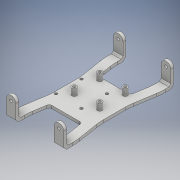
# Autodesk Inventor part: IMU_holder
Saved by Autodesk Inventor 2018 (Build 220112000, 112)
## iProperties
Created: 2018-07-18
Part Number: IMU_holder
Material: Generic
Document SubType Name: Modeling
Designer: Tsche
Density: 1 g/cm^3
Appearance: Default
Author: Tsche
Autodesk Inventor part; units mm, degrees
note: some values were not read from the file. Chosen so that the rebuilt part matches the saved one: direction of "Hole1".
ref_plane "YZ Plane" through (0, 0, 0) normal (1, 0, 0) x (0, 1, 0)
ref_plane "XZ Plane" through (0, 0, 0) normal (0, 1, 0) x (-1, 0, 0)
ref_plane "XY Plane" through (0, 0, 0) normal (0, 0, 1) x (1, 0, 0)
sketch "Sketch1" plane through (0, 0, 0) normal (0, 0, 1) x (1, 0, 0)
  line L0 (-22.86, 13.96) -> (3.81, 13.96) construction
  line L1 (3.81, 13.96) -> (3.81, -12.71) construction
  line L2 (3.81, -12.71) -> (-22.86, -12.71) construction
  line L3 (-22.86, -12.71) -> (-22.86, 13.96) construction
  line L4 (3.81, 0) -> (0, 0) construction
  line L5 (0, 0) -> (0, 13.96) construction
  circle A0 centre (-22.86, 13.96) radius 1.4
  circle A1 centre (3.81, 13.96) radius 1.4
  circle A2 centre (-22.86, -12.71) radius 1.4
  circle A3 centre (3.81, -12.71) radius 1.4
  line L6 (13.96, 22.86) -> (13.96, -3.81) construction
  line L7 (13.96, -3.81) -> (-12.71, -3.81) construction
  line L8 (-12.71, -3.81) -> (-12.71, 22.86) construction
  line L9 (-12.71, 22.86) -> (13.96, 22.86) construction
  line L10 (0, -3.81) -> (0, 0) construction
  line L11 (0, 0) -> (13.96, 0) construction
  circle A4 centre (13.96, 22.86) radius 1.4
  circle A5 centre (13.96, -3.81) radius 1.4
  circle A6 centre (-12.71, 22.86) radius 1.4
  circle A7 centre (-12.71, -3.81) radius 1.4
  line L12 (-30, -57.5) -> (-20, -57.5)
  line L13 (-25, -57.5) -> (-25, -66.2075) construction
  line L14 (25, -57.5) -> (25, -66.2075) construction
  line L15 (0, 215.5444) -> (0, -197.4509) construction
  line L16 (-25.36, 15.21) -> (-25.36, -15.21)
  line L17 (-16.9679, 25.36) -> (16.9679, 25.36)
  line L18 (-30, -57.5) -> (-30, -54.5)
  line L19 (-30, -54.5) -> (30, -54.5) construction
  line L20 (30, -54.5) -> (30, -57.5)
  line L21 (-30, -54.5) -> (-30, -44.5)
  line L22 (-30, -44.5) -> (-25.36, -15.21)
  line L23 (30, -54.5) -> (30, -44.5)
  line L24 (30, -44.5) -> (25.36, -15.21)
  line L25 (25.36, 15.21) -> (25.36, -15.21)
  line L26 (-42, 0) -> (42, 0) construction
  line L27 (-30, 57.5) -> (-20, 57.5)
  line L28 (-25, 57.5) -> (-25, 66.2075) construction
  line L29 (25, 57.5) -> (25, 66.2075) construction
  line L30 (-30, 57.5) -> (-30, 54.5)
  line L31 (-30, 54.5) -> (30, 54.5) construction
  line L32 (30, 54.5) -> (30, 57.5)
  line L33 (-30, 54.5) -> (-30, 44.5)
  line L34 (-30, 44.5) -> (-25.36, 15.21)
  line L35 (30, 44.5) -> (25.36, 15.21)
  line L36 (30, 54.5) -> (30, 44.5)
  line L37 (-16.9679, 25.36) -> (-20, 44.5)
  line L38 (-20, 44.5) -> (-20, 54.5)
  line L39 (16.9679, 25.36) -> (20, 44.5)
  line L40 (20, 44.5) -> (20, 54.5)
  line L41 (0, -215.5444) -> (0, 197.4509) construction
  line L42 (-16.9679, -25.36) -> (16.9679, -25.36)
  line L43 (-16.9679, -25.36) -> (-20, -44.5)
  line L44 (-20, -44.5) -> (-20, -54.5)
  line L45 (16.9679, -25.36) -> (20, -44.5)
  line L46 (20, -44.5) -> (20, -54.5)
  line L47 (-20, -54.5) -> (-20, -57.5)
  line L48 (20, -54.5) -> (20, -57.5)
  line L49 (-20, 54.5) -> (-20, 57.5)
  line L50 (20, 54.5) -> (20, 57.5)
  line L51 (-20, -57.5) -> (20, -57.5) construction
  line L52 (20, -57.5) -> (30, -57.5)
  line L53 (-20, 57.5) -> (20, 57.5) construction
  line L54 (20, 57.5) -> (30, 57.5)
  dimension "d0" = 26.67
  dimension "d1" = 13.96
  dimension "d2" = 3.81
  dimension "d3" = 2.8
  dimension "d6" = 90
  dimension "d8" = 57.5
  dimension "d10" = 50
  dimension "d11" = 5
  dimension "d12" = 2.5
  dimension "d13" = 2.5
  dimension "d16" = 3
  dimension "d17" = 2.5
  dimension "d18" = 10
  dimension "d19" = 10
  dimension "d35" = 5
  constraints: 106 end point, 28 symmetric about line, 13 point on line, 11 coincident, 11 perpendicular, 8 centre point, 7 horizontal, 5 vertical, 4 midpoint, 3 equal radius, 3 parallel, 23 other
  measures "d0" distance of L2.end L0.start
  measures "d1" distance of L4.end L5.end
  measures "d2" distance of L4.start L4.end
  measures "d3" diameter of A0
  measures "d8" distance from line of point (0, 0) L12
  measures "d10" distance between parallel lines of L13 L14
  measures "d11" distance from line of L20.end L14
  measures "d12" distance between parallel lines of L16 L3
  measures "d13" distance from line of L6.start L17
  measures "d16" distance of L12.start L18.end
  measures "d17" horizontal distance of L2.end L16.end
  measures "d18" distance of L18.end L21.end
  measures "d19" distance of L37.end L38.end
  measures "d35" distance between parallel lines of L13 L44
extrude "Extrusion1" add sketch "Sketch1" along normal blind 3
sketch "Sketch2" plane through (0, 0, 3) normal (0, 0, 1) x (1, 0, 0)
  circle A0 centre (-22.86, 13.96) radius 1.4 projected
  circle A1 centre (-12.71, 22.86) radius 1.4 projected
  circle A2 centre (3.81, 13.96) radius 1.4 projected
  circle A3 centre (13.96, 22.86) radius 1.4 projected
  circle A4 centre (13.96, -3.81) radius 1.4 projected
  circle A5 centre (3.81, -12.71) radius 1.4 projected
  circle A6 centre (-12.71, -3.81) radius 1.4 projected
  circle A7 centre (-22.86, -12.71) radius 1.4 projected
  circle A8 centre (-22.86, 13.96) radius 2.5
  line L0 (-25.36, 15.21) -> (-25.36, -15.21) construction
  circle A9 centre (-22.86, -12.71) radius 2.5
  circle A10 centre (-12.71, -3.81) radius 2.5
  circle A11 centre (-12.71, 22.86) radius 2.5
  circle A12 centre (3.81, 13.96) radius 2.5
  circle A13 centre (13.96, 22.86) radius 1.4 projected
  circle A14 centre (13.96, 22.86) radius 2.5
  circle A15 centre (13.96, -3.81) radius 2.5
  circle A16 centre (3.81, -12.71) radius 2.5
  point P0 (0, 0)
  constraints: 8 centre point, 8 coincident, 6 equal radius, 2 tangent
extrude "Extrusion2" add sketch "Sketch2" along normal blind 7 contours A10 | A11 | A14 | A15
sketch "Sketch3" plane through (0, 0, 3) normal (0, 0, 1) x (1, 0, 0)
  line L0 (-30, -54.5) -> (30, -54.5) construction
  line L1 (-30, -57.5) -> (-20, -57.5) construction
  line L2 (-20, -54.5) -> (-20, -57.5) construction
  line L3 (-30, -44.5) -> (-30, -57.5) construction
  line L4 (30, -57.5) -> (30, -44.5) construction
  line L5 (20, -44.5) -> (20, -57.5) construction
  line L6 (20, -57.5) -> (30, -57.5) construction
  line L7 (-30, -54.5) -> (-20, -54.5)
  line L8 (-20, -54.5) -> (-20, -57.5)
  line L9 (-20, -57.5) -> (-30, -57.5)
  line L10 (-30, -57.5) -> (-30, -54.5)
  line L11 (20, -57.5) -> (30, -57.5) projected
  line L12 (20, -57.5) -> (30, -57.5)
  line L13 (30, -57.5) -> (30, -54.5)
  line L14 (30, -54.5) -> (20, -54.5)
  line L15 (20, -54.5) -> (20, -57.5)
  line L16 (-42, 0) -> (42, 0) construction
  line L17 (-30, 57.5) -> (-20, 57.5) construction
  line L18 (-20, 54.5) -> (-20, 57.5) construction
  line L19 (20, 57.5) -> (30, 57.5) construction
  line L20 (-30, 54.5) -> (-20, 54.5)
  line L21 (-20, 54.5) -> (-20, 57.5)
  line L22 (-20, 57.5) -> (-30, 57.5)
  line L23 (-30, 57.5) -> (-30, 54.5)
  line L24 (20, 57.5) -> (30, 57.5)
  line L25 (20, 57.5) -> (30, 57.5)
  line L26 (30, 57.5) -> (30, 54.5)
  line L27 (30, 54.5) -> (20, 54.5)
  line L28 (20, 54.5) -> (20, 57.5)
  point P0 (0, 0)
  constraints: 40 end point, 13 symmetric about line, 4 parallel, 2 horizontal, 2 perpendicular
extrude "Extrusion3" add sketch "Sketch3" along normal blind 20
hole "Hole1" at (-25, -57.5, 18) direction (0, 1, 0) diameter 2.8 end up to surface
mirror "Mirror1" about plane through (0, 0, 0) normal (1, 0, 0) of "Hole1"
mirror "Mirror2" about plane through (0, 0, 0) normal (0, 1, 0) of "Hole1", "Mirror1"
fillet "Fillet1" radius 50 12 edges at (-30, 44.5, 1.5) (-25.36, 15.21, 1.5) (-30, -44.5, 1.5) (-25.36, -15.21, 1.5) (-20, 44.5, 1.5) (20, 44.5, 1.5) (30, 44.5, 1.5) (25.36, 15.21, 1.5) (25.36, -15.21, 1.5) (20, -44.5, 1.5) (-20, -44.5, 1.5) (30, -44.5, 1.5)
fillet "Fillet2" radius 3 4 edges at (-16.9679, 25.36, 1.5) (16.9679, 25.36, 1.5) (-16.9679, -25.36, 1.5) (16.9679, -25.36, 1.5)
chamfer "Chamfer1" distance 2 angle 45 4 edges at (-25, 54.5, 3) (25, 54.5, 3) (-25, -54.5, 3) (25, -54.5, 3)
chamfer "Chamfer2" distance 3 angle 45 4 edges at (25, 57.5, 0) (-25, 57.5, 0) (-25, -57.5, 0) (25, -57.5, 0)
fillet "Fillet3" radius 5 8 edges at (30, 56, 23) (20, 56, 23) (-20, 56, 23) (-30, 56, 23) (30, -56, 23) (20, -56, 23) (-20, -56, 23) (-30, -56, 23)
body "Solid1"
